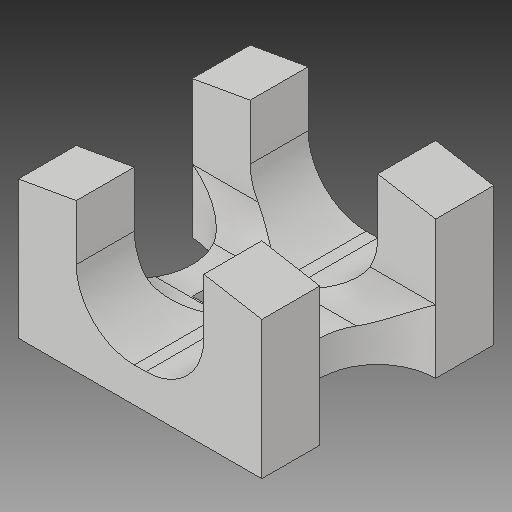
# Autodesk Inventor part: Foot_Ankl_Connector
Saved by Autodesk Inventor 2019 (Build 230136000, 136)
## iProperties
Created: 2018-06-02
Part Number: Foot_Ankl_Connector
Material: Generic
Document SubType Name: Modeling
Designer: Till
Density: 1 g/cm^3
Appearance: Default
Mass: 130.337 g
Surface Area: 276.644 cm^2
Volume: 130.337 cm^3
Author: Till
Autodesk Inventor part; units mm, degrees
ref_plane "YZ Plane" through (0, 0, 0) normal (1, 0, 0) x (0, 1, 0)
ref_plane "XZ Plane" through (0, 0, 0) normal (0, 1, 0) x (-1, 0, 0)
ref_plane "XY Plane" through (0, 0, 0) normal (0, 0, 1) x (1, 0, 0)
sketch "Sketch1" plane through (0, 0, 0) normal (0, 0, 1) x (1, 0, 0)
  line L0 (-42, 0) -> (42, 0)
  line L1 (42, 0) -> (42, -12)
  line L2 (42, -12) -> (-42, -12)
  line L3 (-42, -12) -> (-42, 0)
  line L4 (0, -14.4) -> (0, 2.4) projected
  point P0 (0, 0)
  dimension "d0" = 84
  dimension "d1" = 12
  constraints: 8 end point, 2 parallel, 1 horizontal, 1 midpoint, 1 perpendicular, 1 other
  measures "d0" distance of L1.end L2.end
  measures "d1" distance of L2.end L0.start
extrude "Extrusion1" add sketch "Sketch1" along normal mid plane 80
sketch "Sketch2" plane through (-42, 0, 40) normal (0, 1, 0) x (1, 0, 0)
  line L0 (29.5, 49.5) -> (54.5, 49.5)
  line L1 (54.5, 49.5) -> (54.5, 30.5)
  line L2 (54.5, 30.5) -> (29.5, 30.5)
  line L3 (29.5, 30.5) -> (29.5, 49.5)
  line L4 (-16.8, 40) -> (100.8, 40) projected
  line L5 (42, 96) -> (42, -16) projected
  point P0 (42, 40)
  dimension "d4" = 19
  dimension "d5" = 25
  constraints: 8 end point, 2 parallel, 1 horizontal, 1 perpendicular, 2 other
  measures "d4" distance of L2.end L0.start
  measures "d5" distance of L0.start L0.end
extrude "Extrusion2" cut sketch "Sketch2" against normal blind 7
sketch "Sketch3" plane through (-42, 0, 40) normal (0, 1, 0) x (1, 0, 0)
  point P0 (42, 40)
  point P1 (42, 40)
  constraints: 1 coincident
hole "Hole1" at (0, 0, 0) direction (0, -1, 0) diameter 12 end through all
sketch "Sketch5" plane through (0, 0, 0) normal (0, 0, 1) x (1, 0, 0)
  circle A0 centre (0, 43) radius 10.1 projected
  line L0 (0, 43) -> (42, 35.5943)
  line L1 (42, 0) -> (-42, 0) projected
  line L2 (42, 35.5943) -> (42, 0)
  line L3 (22, 0) -> (22, 39.1208)
  line L4 (22, 0) -> (42, 0)
  line L5 (0, -10.62) -> (0, 63.72) projected
  line L6 (0, 43) -> (-42, 35.5943)
  line L7 (-42, 0) -> (42, 0)
  line L8 (-42, 35.5943) -> (-42, 0)
  line L9 (-22, 0) -> (-22, 39.1208)
  point P0 (0, 0)
  dimension "d23" = 22
  dimension "d24" = 42
  dimension "d29" = 10
  constraints: 16 end point, 6 point on line, 6 symmetric about line, 1 collinear, 1 parallel, 1 perpendicular
  measures "d23" distance from line of L3 point (0, 0)
  measures "d24" distance from line of L2 point (0, 0)
  measures "d29" angle of L1 L0
extrude "Extrusion3" add sketch "Sketch5" along normal mid plane 80 contours L0 L2 L1 L3 | L9 L1 L8 L6
sketch "Sketch7" plane through (42, -12, 40) normal (1, 0, 0) x (0, 0, -1)
  line L0 (20, 0) -> (60, 0)
  line L1 (60, 0) -> (60, 51.1208)
  line L2 (60, 51.1208) -> (20, 51.1208)
  line L3 (20, 51.1208) -> (20, 0)
  line L4 (80, 47.5943) -> (80, 0) projected
  line L5 (0, 0) -> (0, 47.5943) projected
  line L6 (0, 0) -> (80, 0) projected
  line L7 (80, 51.1208) -> (0, 51.1208) projected
  point P0 (40, 12)
  dimension "d35" = 20
  dimension "d36" = 20
  dimension "d37" = 0
  dimension "d38" = 0
  constraints: 8 end point, 2 parallel, 1 horizontal, 1 perpendicular
  measures "d35" distance between parallel lines of L4 L1
  measures "d36" distance between parallel lines of L5 L3
  measures "d37" distance between parallel lines of L6 L0
  measures "d38" distance between parallel lines of L7 L2
sketch "Sketch8" plane through (-42, -12, -40) normal (-1, 0, 0) x (0, 0, 1)
  line L0 (80, 0) -> (0, 0) projected
  line L1 (20, 51.1208) -> (60, 51.1208)
  line L2 (60, 51.1208) -> (60, 0)
  line L3 (60, 0) -> (20, 0)
  line L4 (20, 0) -> (20, 51.1208)
  line L5 (80, 47.5943) -> (80, 0) projected
  line L6 (0, 0) -> (0, 47.5943) projected
  line L7 (80, 51.1208) -> (0, 51.1208) projected
  point P0 (40, 12)
  dimension "d39" = 20
  dimension "d40" = 20
  dimension "d41" = 0
  constraints: 8 end point, 2 parallel, 1 horizontal, 1 perpendicular, 1 point on line
  measures "d39" distance between parallel lines of L5 L2
  measures "d40" distance between parallel lines of L6 L4
  measures "d41" distance between parallel lines of L7 L1
extrude "Extrusion5" cut sketch "Sketch8" against normal blind 20
extrude "Extrusion6" cut sketch "Sketch7" against normal blind 20
fillet "Fillet1" radius 20 8 edges at (-22, -6, -20) (-22, -6, 20) (-22, 0, -30) (22, 0, -30) (22, -6, 20) (22, -6, -20) (22, 0, 30) (-22, 0, 30)
fillet "Fillet2" radius 10 8 edges at (31.9999, 0, 20) (12, 0, 20) (-12, 0, 20) (-31.9999, 0, 20) (31.9999, 0, -20) (12, 0, -20) (-12, 0, -20) (-31.9999, 0, -20)
body "Solid1"
